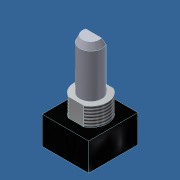
# Autodesk Inventor part: Potentiomètre
Saved by Autodesk Inventor 2015 SP2 (Build 190223200, 223)
## iProperties
Created: 2017-10-30
Part Number: Potentiomètre
Material: Générique
Document SubType Name: Modeling
Designer: Alexandre.PICOTTE
Density: 1 g/cm^3
Appearance: Vert turquoise
Author: Alexandre.PICOTTE
Autodesk Inventor part; units mm, degrees
ref_plane "YZ Plane" through (0, 0, 0) normal (1, 0, 0) x (0, 1, 0)
ref_plane "XZ Plane" through (0, 0, 0) normal (0, 1, 0) x (-1, 0, 0)
ref_plane "XY Plane" through (0, 0, 0) normal (0, 0, 1) x (1, 0, 0)
sketch "Esquisse1" plane through (0, 0, 0) normal (0, 0, 1) x (1, 0, 0)
  circle A0 centre (0, 0) radius 3
  dimension "d0" = 6
  constraints: 1 centre point, 1 coincident
  measures "d0" diameter of A0
extrude "Extrusion1" add sketch "Esquisse1" along normal blind 13.4
sketch "Esquisse2" plane through (0, 0, 13.4) normal (0, 0, 1) x (1, 0, 0)
  line L0 (-3, 3) -> (3, 3)
  line L1 (3, 3) -> (3, 1.5)
  line L2 (3, 1.5) -> (-3, 1.5)
  line L3 (-3, 1.5) -> (-3, 3)
  circle A0 centre (0, 0) radius 3 projected
  dimension "d3" = 1.5
  constraints: 8 end point, 3 tangent, 2 parallel, 1 horizontal, 1 perpendicular
  measures "d3" distance of L0.end L1.end
extrude "Extrusion2" cut sketch "Esquisse2" against normal blind 11.8 contours L0 A0 L2 L3 | L0 L1 L2 A0 | A0 L2 picked at (-0.7431, 1.6691)
sketch "Esquisse4" plane through (0, 0, 0) normal (0, 0, -1) x (-1, 0, 0)
  line L0 (-2.0616, 4) -> (2.0616, 4)
  line L1 (2.0616, -4) -> (-2.0616, -4)
  line L2 (0, -6.3) -> (0, 6.3) construction
  line L3 (6.3, 0) -> (-6.3, 0) construction
  circle A0 centre (0, 0) radius 4.5
  point P0 (-4, 2.0616)
  point P1 (4, -2.0616)
  point P2 (-4, -2.0616)
  point P3 (4, 2.0616)
  dimension "d10" = 9
  dimension "d12" = 8
  constraints: 4 end point, 1 coincident, 1 horizontal, 1 parallel, 11 other
  measures "d12" distance between parallel lines of L1 L0
extrude "Extrusion4" add sketch "Esquisse4" along normal blind 5 contours L0 A0 L1
thread "Filetage1" size "M9x0.75" class "6g" standard "ANSI Metric M Profile" full length
thread "Filetage3" size "M9x0.75" class "6g" standard "ANSI Metric M Profile" full length
sketch "Esquisse5" plane through (0, 0, -5) normal (0, 0, -1) x (-1, 0, 0)
  line L0 (6.5, 6.635) -> (-6.03, 6.635)
  line L1 (-6.03, 6.635) -> (-6.03, -6.635)
  line L2 (-6.03, -6.635) -> (6.5, -6.635)
  line L3 (6.5, -6.635) -> (6.5, 6.635)
  line L4 (9.006, 0) -> (-8.536, 0) construction
  line L5 (0, -9.289) -> (0, 9.289) construction
  point P0 (0, 0)
  dimension "d24" = 12.53
  dimension "d25" = 6.5
  dimension "d26" = 13.27
  constraints: 8 end point, 2 parallel, 1 horizontal, 1 perpendicular, 1 other
  measures "d24" distance of L0.start L0.end
  measures "d25" distance from line of point (0, 0) L3
  measures "d26" distance of L2.end L0.start
extrude "Extrusion5" add sketch "Esquisse5" along normal blind 7.5
chamfer "Chanfrein1" distance 0.75 distance2 1.68 1 edges at (0, 1.5, 13.4) measured on face at (0, 1, 13.4)
chamfer "Chanfrein2" distance 0.75 distance2 1.68 2 edges at (-0.378, -2.9761, 13.4) (2.9761, 0.378, 13.4) measured on face at (2.4801, 0.315, 13.4) measured on face at (-0.315, -2.4801, 13.4)
